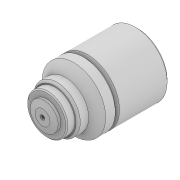
# Autodesk Inventor part: 210505 - Zeiss x100 objective mockup
Saved by Autodesk Inventor 2020 (Build 240168000, 168)
## iProperties
Created: 2021-05-05
Part Number: 210505 - Zeiss x100 objective mockup
Material: Generic
Document SubType Name: Modeling
Designer: Ralf
Density: 1 g/cm^3
Appearance: Default
Author: Ralf
Autodesk Inventor part; units mm, degrees
ref_plane "YZ Plane" through (0, 0, 0) normal (1, 0, 0) x (0, 1, 0)
ref_plane "XZ Plane" through (0, 0, 0) normal (0, 1, 0) x (-1, 0, 0)
ref_plane "XY Plane" through (0, 0, 0) normal (0, 0, 1) x (1, 0, 0)
sketch "Sketch1" plane through (0, 0, 0) normal (0, 0, 1) x (1, 0, 0)
  circle A0 centre (0, 0) radius 15
  dimension "d0" = 30
  constraints: 1 centre point, 1 coincident
  measures "d0" diameter of A0
extrude "Extrusion1" add sketch "Sketch1" along normal blind 24.5
chamfer "Chamfer1" distance 1 angle 45 2 edges at (-15, 0, 24.5) (-15, 0, 0)
sketch "Sketch2" plane through (0, 0, 24.5) normal (0, 0, 1) x (1, 0, 0)
  circle A0 centre (0, 0) radius 15
  dimension "d6" = 30
  constraints: 1 centre point, 1 coincident
  measures "d6" diameter of A0
extrude "Extrusion2" add sketch "Sketch2" along normal blind 5.5
chamfer "Chamfer2" distance 1 angle 45 1 edges at (-15, 0, 24.5)
sketch "Sketch3" plane through (0, 0, 30) normal (0, 0, 1) x (1, 0, 0)
  circle A0 centre (0, 0) radius 11
  dimension "d12" = 22
  constraints: 1 centre point, 1 coincident
  measures "d12" diameter of A0
extrude "Extrusion3" add sketch "Sketch3" along normal blind 4
chamfer "Chamfer3" distance 4 angle 45 1 edges at (-11, 0, 30)
sketch "Sketch4" plane through (0, 0, 34) normal (0, 0, 1) x (1, 0, 0)
  circle A0 centre (0, 0) radius 11
  dimension "d18" = 22
  constraints: 1 centre point, 1 coincident
  measures "d18" diameter of A0
extrude "Extrusion4" add sketch "Sketch4" along normal blind 5
sketch "Sketch5" plane through (0, 0, 39) normal (0, 0, 1) x (1, 0, 0)
  circle A0 centre (0, 0) radius 9.5
  dimension "d21" = 19
  constraints: 1 centre point, 1 coincident
  measures "d21" diameter of A0
extrude "Extrusion5" add sketch "Sketch5" along normal blind 3.8
chamfer "Chamfer4" distance 1 angle 45 1 edges at (-11, 0, 39)
sketch "Sketch6" plane through (0, 0, 42.8) normal (0, 0, 1) x (1, 0, 0)
  circle A0 centre (0, 0) radius 6.6
  dimension "d27" = 13.2
  constraints: 1 centre point, 1 coincident
  measures "d27" diameter of A0
extrude "Extrusion6" add sketch "Sketch6" along normal blind 0.75
sketch "Sketch7" plane through (0, 0, 43.55) normal (0, 0, 1) x (1, 0, 0)
  circle A0 centre (0, 0) radius 3.55
  dimension "d30" = 7.1
  constraints: 1 centre point, 1 coincident
  measures "d30" diameter of A0
extrude "Extrusion7" add sketch "Sketch7" along normal blind 1.25
sketch "Sketch8" plane through (0, 0, 0) normal (0, 1, 0) x (-1, 0, 0)
  line L0 (3.55, 44.8) -> (-3.55, 44.8) projected
  line L1 (3.55, 44.8) -> (6.6, 44.0124)
  line L2 (3.55, 44.8) -> (6.7001, 44.8) construction
  line L3 (6.6, 43.55) -> (-6.6, 43.55) projected
  line L4 (6.6, 44.0124) -> (6.6, 43.55)
  line L5 (6.6, 43.55) -> (3.55, 43.55)
  line L6 (3.55, 43.55) -> (3.55, 44.8) projected
  line L7 (3.55, 44.8) -> (3.55, 43.7812)
  line L8 (0, -8.96) -> (0, 53.76) projected
  point P0 (0, 0)
  dimension "d33" = 14.48
  constraints: 10 end point, 2 perpendicular, 2 point on line, 1 equal length, 1 horizontal
  measures "d33" angle of L1 L2
revolve "Revolution1" add sketch "Sketch8" angle 360 about axis through (0, 0, -10) along (0, 0, 1) contours L1 L4 L3 L6
sketch "Sketch9" plane through (0, 0, 44.8) normal (0, 0, 1) x (1, 0, 0)
  circle A0 centre (0, 0) radius 1
  dimension "d35" = 2
  constraints: 1 centre point, 1 coincident
  measures "d35" diameter of A0
extrude "Extrusion8" cut sketch "Sketch9" against normal blind 50
sketch "Sketch10" plane through (0, 0, 0) normal (0, 0, -1) x (-1, 0, 0)
  circle A0 centre (0, 0) radius 2
  dimension "d38" = 4
  constraints: 1 centre point, 1 coincident
  measures "d38" diameter of A0
extrude "Extrusion9" cut sketch "Sketch10" against normal blind 20
chamfer "Chamfer5" distance 0.5 angle 45 1 edges at (-9.5, 0, 42.8)
body "Solid1"
